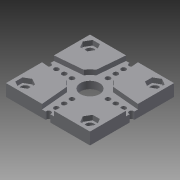
# Autodesk Inventor part: handPivot
Saved by Autodesk Inventor 2015 (Build 190159000, 159)
## iProperties
Created: 2016-10-16
Part Number: handPivot
Material: Generic
Document SubType Name: Modeling
Designer: Bardo91
Density: 1 g/cm^3
Appearance: Default
Author: Bardo91
Autodesk Inventor part; units mm, degrees
ref_plane "YZ Plane" through (0, 0, 0) normal (1, 0, 0) x (0, 1, 0)
ref_plane "XZ Plane" through (0, 0, 0) normal (0, 1, 0) x (-1, 0, 0)
ref_plane "XY Plane" through (0, 0, 0) normal (0, 0, 1) x (1, 0, 0)
sketch "Sketch1" plane through (0, 0, 0) normal (0, 0, 1) x (1, 0, 0)
  line L0 (0, 0) -> (0, 17.5)
  line L1 (0, 17.5) -> (-17.5, 17.5)
  line L2 (-17.5, 17.5) -> (-17.5, -17.5)
  line L3 (-17.5, -17.5) -> (17.5, -17.5)
  line L4 (17.5, -17.5) -> (17.5, 17.5)
  line L5 (17.5, 17.5) -> (0, 17.5)
  line L6 (-17.5, 17.5) -> (-17.5, 13.5)
  line L7 (-17.5, 13.5) -> (-13.5, 13.5)
  circle A0 centre (-13.5, 13.5) radius 1.75
  circle A1 centre (-13.5, -13.5) radius 1.75
  circle A2 centre (13.5, -13.5) radius 1.75
  circle A3 centre (13.5, 13.5) radius 1.75
  dimension "d0" = 17.5
  dimension "d1" = 17.5
  dimension "d2" = 35
  dimension "d3" = 35
  dimension "d4" = 4
  dimension "d5" = 4
  dimension "d6" = 3.5
  dimension "d9" = 360
  constraints: 16 end point, 6 perpendicular, 4 centre point, 2 point on line, 1 coincident, 1 vertical, 9 other
  measures "d0" distance of L0.start L0.end
  measures "d1" distance of L0.end L1.end
  measures "d2" distance of L1.end L2.end
  measures "d3" distance of L2.end L3.end
  measures "d4" distance of L1.end L6.end
  measures "d5" distance of L6.end L7.end
  measures "d6" diameter of A0
extrude "Extrusion1" add sketch "Sketch1" along normal blind 5
sketch "Sketch2" plane through (0, 0, 5) normal (0, 0, 1) x (1, 0, 0)
  line L0 (0, 0) -> (0, 17)
  line L1 (0, 0) -> (0, -17)
  arc A0 (2.4898, 17.2253) -> (-2.4898, 17.2253) centre (0, 17) ccw
  circle A1 centre (0, -17) radius 2.5
  line L2 (0, 0) -> (7, 0) construction
  line L3 (3.5, 6.0622) -> (2.4898, 17.2253)
  line L4 (-3.5, 6.0622) -> (-2.4898, 17.2253)
  arc A2 (-17.2253, 2.4898) -> (-17.2253, -2.4898) centre (-17, 0) ccw
  line L5 (-6.0622, 3.5) -> (-17.2253, 2.4898)
  line L6 (-6.0622, -3.5) -> (-17.2253, -2.4898)
  arc A3 (-2.4898, -17.2253) -> (2.4898, -17.2253) centre (0, -17) ccw
  line L7 (-3.5, -6.0622) -> (-2.4898, -17.2253)
  line L8 (3.5, -6.0622) -> (2.4898, -17.2253)
  arc A4 (17.2253, -2.4898) -> (17.2253, 2.4898) centre (17, 0) ccw
  line L9 (6.0622, -3.5) -> (17.2253, -2.4898)
  line L10 (6.0622, 3.5) -> (17.2253, 2.4898)
  arc A5 (-6.0622, -3.5) -> (-3.5, -6.0622) centre (0, 0) ccw
  arc A6 (3.5, -6.0622) -> (6.0622, -3.5) centre (0, 0) ccw
  arc A7 (6.0622, 3.5) -> (3.5, 6.0622) centre (0, 0) ccw
  arc A8 (-3.5, 6.0622) -> (-6.0622, 3.5) centre (0, 0) ccw
  dimension "d21" = 360
  dimension "d13" = 17
  dimension "d14" = 17
  dimension "d15" = 5
  dimension "d16" = 5
  constraints: 22 end point, 16 point on circle, 9 centre point, 3 coincident, 2 tangent, 2 vertical, 1 horizontal, 33 other
  measures "d13" distance of L0.start L0.end
  measures "d14" distance of L0.start L1.end
  measures "d15" diameter of A0
  measures "d16" diameter of A1
extrude "Extrusion2" cut sketch "Sketch2" against normal blind 2
sketch "Sketch3" plane through (0, 0, 3) normal (0, 0, 1) x (1, 0, 0)
  circle A0 centre (0, 0) radius 4
  dimension "d25" = 8
  constraints: 1 centre point, 1 coincident
  measures "d25" diameter of A0
extrude "Extrusion3" cut sketch "Sketch3" against normal through all
sketch "Sketch4" plane through (0, 0, 3) normal (0, 0, 1) x (1, 0, 0)
  line L0 (0, 0) -> (0, 7.5)
  circle A0 centre (0, 7.5) radius 1
  circle A1 centre (0, 10.75) radius 1
  circle A2 centre (0, 14) radius 1
  circle A3 centre (0, 17.25) radius 1
  circle A4 centre (-7.5, 0) radius 1
  circle A5 centre (-10.75, 0) radius 1
  circle A6 centre (-14, 0) radius 1
  circle A7 centre (-17.25, 0) radius 1
  circle A8 centre (0, -7.5) radius 1
  circle A9 centre (0, -10.75) radius 1
  circle A10 centre (0, -14) radius 1
  circle A11 centre (0, -17.25) radius 1
  circle A12 centre (7.5, 0) radius 1
  circle A13 centre (10.75, 0) radius 1
  circle A14 centre (14, 0) radius 1
  circle A15 centre (17.25, 0) radius 1
  dimension "d28" = 7.5
  dimension "d29" = 2
  dimension "d32" = 3.25
  dimension "d39" = 360
  constraints: 16 centre point, 2 end point, 2 vertical, 1 coincident, 39 other
  measures "d28" distance of L0.start L0.end
  measures "d29" diameter of A0
  measures "d32" distance of A0.centre A1.centre
extrude "Extrusion4" cut sketch "Sketch4" against normal through all
sketch "Sketch5" plane through (0, 0, 5) normal (0, 0, 1) x (1, 0, 0)
  circle A0 centre (-13.5, 13.5) radius 1.75 projected
  line L0 (-13.5, 13.5) -> (-10.5, 13.5)
  line L1 (-10.5, 13.5) -> (-12, 16.0981)
  line L2 (-12, 16.0981) -> (-13.5, 13.5)
  line L3 (-13.5, 13.5) -> (-12, 16.0981)
  line L4 (-12, 16.0981) -> (-15, 16.0981)
  line L5 (-15, 16.0981) -> (-13.5, 13.5)
  line L6 (-13.5, 13.5) -> (-15, 16.0981)
  line L7 (-15, 16.0981) -> (-16.5, 13.5)
  line L8 (-16.5, 13.5) -> (-13.5, 13.5)
  line L9 (-13.5, 13.5) -> (-16.5, 13.5)
  line L10 (-16.5, 13.5) -> (-15, 10.9019)
  line L11 (-15, 10.9019) -> (-13.5, 13.5)
  line L12 (-13.5, 13.5) -> (-15, 10.9019)
  line L13 (-15, 10.9019) -> (-12, 10.9019)
  line L14 (-12, 10.9019) -> (-13.5, 13.5)
  line L15 (-13.5, 13.5) -> (-12, 10.9019)
  line L16 (-12, 10.9019) -> (-10.5, 13.5)
  line L17 (-10.5, 13.5) -> (-13.5, 13.5)
  line L18 (-13.5, -13.5) -> (-13.5, -10.5)
  line L19 (-13.5, -10.5) -> (-16.0981, -12)
  line L20 (-16.0981, -12) -> (-13.5, -13.5)
  line L21 (-16.0981, -15) -> (-13.5, -13.5)
  line L22 (-16.0981, -12) -> (-16.0981, -15)
  line L23 (-13.5, -13.5) -> (-16.0981, -12)
  line L24 (-13.5, -16.5) -> (-13.5, -13.5)
  line L25 (-16.0981, -15) -> (-13.5, -16.5)
  line L26 (-13.5, -13.5) -> (-16.0981, -15)
  line L27 (-10.9019, -15) -> (-13.5, -13.5)
  line L28 (-13.5, -16.5) -> (-10.9019, -15)
  line L29 (-13.5, -13.5) -> (-13.5, -16.5)
  line L30 (-10.9019, -12) -> (-13.5, -13.5)
  line L31 (-10.9019, -15) -> (-10.9019, -12)
  line L32 (-13.5, -13.5) -> (-10.9019, -15)
  line L33 (-13.5, -10.5) -> (-13.5, -13.5)
  line L34 (-10.9019, -12) -> (-13.5, -10.5)
  line L35 (-13.5, -13.5) -> (-10.9019, -12)
  line L36 (13.5, -13.5) -> (10.5, -13.5)
  line L37 (10.5, -13.5) -> (12, -16.0981)
  line L38 (12, -16.0981) -> (13.5, -13.5)
  line L39 (15, -16.0981) -> (13.5, -13.5)
  line L40 (12, -16.0981) -> (15, -16.0981)
  line L41 (13.5, -13.5) -> (12, -16.0981)
  line L42 (16.5, -13.5) -> (13.5, -13.5)
  line L43 (15, -16.0981) -> (16.5, -13.5)
  line L44 (13.5, -13.5) -> (15, -16.0981)
  line L45 (15, -10.9019) -> (13.5, -13.5)
  line L46 (16.5, -13.5) -> (15, -10.9019)
  line L47 (13.5, -13.5) -> (16.5, -13.5)
  line L48 (12, -10.9019) -> (13.5, -13.5)
  line L49 (15, -10.9019) -> (12, -10.9019)
  line L50 (13.5, -13.5) -> (15, -10.9019)
  line L51 (10.5, -13.5) -> (13.5, -13.5)
  line L52 (12, -10.9019) -> (10.5, -13.5)
  line L53 (13.5, -13.5) -> (12, -10.9019)
  line L54 (13.5, 13.5) -> (13.5, 10.5)
  line L55 (13.5, 10.5) -> (16.0981, 12)
  line L56 (16.0981, 12) -> (13.5, 13.5)
  line L57 (16.0981, 15) -> (13.5, 13.5)
  line L58 (16.0981, 12) -> (16.0981, 15)
  line L59 (13.5, 13.5) -> (16.0981, 12)
  line L60 (13.5, 16.5) -> (13.5, 13.5)
  line L61 (16.0981, 15) -> (13.5, 16.5)
  line L62 (13.5, 13.5) -> (16.0981, 15)
  line L63 (10.9019, 15) -> (13.5, 13.5)
  line L64 (13.5, 16.5) -> (10.9019, 15)
  line L65 (13.5, 13.5) -> (13.5, 16.5)
  line L66 (10.9019, 12) -> (13.5, 13.5)
  line L67 (10.9019, 15) -> (10.9019, 12)
  line L68 (13.5, 13.5) -> (10.9019, 15)
  line L69 (13.5, 10.5) -> (13.5, 13.5)
  line L70 (10.9019, 12) -> (13.5, 10.5)
  line L71 (13.5, 13.5) -> (10.9019, 12)
  point P0 (0, 0)
  dimension "d43" = 3
  dimension "d44" = 3
  dimension "d45" = 60
  dimension "d48" = 360
  dimension "d52" = 360
  constraints: 144 end point, 2 coincident, 1 horizontal, 180 other
  measures "d43" distance of L0.start L0.end
  measures "d44" distance of L0.end L1.end
  measures "d45" angle of L1 L0
extrude "Extrusion5" cut sketch "Sketch5" against normal blind 2
body "Solid1"
